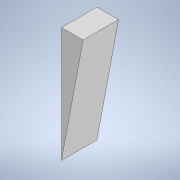
# Autodesk Inventor part: backPlateForLight
Saved by Autodesk Inventor 2021.1 (Build 251245000, 245)
## iProperties
Created: 2020-08-01
Part Number: backPlateForLight
Material: Generic
Document SubType Name: Modeling
Designer: robst
Density: 1 g/cm^3
Appearance: Default
Author: robst
Autodesk Inventor part; units mm, degrees
ref_plane "YZ Plane" through (0, 0, 0) normal (1, 0, 0) x (0, 1, 0)
ref_plane "XZ Plane" through (0, 0, 0) normal (0, 1, 0) x (-1, 0, 0)
ref_plane "XY Plane" through (0, 0, 0) normal (0, 0, 1) x (1, 0, 0)
sketch "Sketch1" plane through (0, 0, 0) normal (0, 0, 1) x (1, 0, 0)
  line L0 (0, 0) -> (0, 82.55)
  line L1 (0, 82.55) -> (15.494, 82.55)
  line L2 (15.494, 82.55) -> (0, 0)
  dimension "d0" = 82.55
  dimension "d1" = 15.494
  constraints: 6 end point, 1 perpendicular, 1 vertical
  measures "d0" distance of L0.start L0.end
  measures "d1" distance of L0.end L1.end
extrude "Extrusion1" add sketch "Sketch1" against normal blind 25.4
sketch "Sketch2" plane through (0, 0, 0) normal (-1, 0, 0) x (0, 0, 1)
  line L0 (-25.4, 82.55) -> (-25.4, 0) projected
  line L1 (-25.4, 62.641) -> (0, 62.641) construction
  line L2 (0, 0) -> (0, 82.55) projected
  line L3 (-14.8227, 65.816) -> (-17.0097, 59.466)
  line L4 (-17.0097, 59.466) -> (-17.9205, 59.466)
  line L5 (-17.9205, 59.466) -> (-20.1075, 65.816)
  line L6 (-20.1075, 65.816) -> (-19.2018, 65.816)
  line L7 (-19.2018, 65.816) -> (-17.4419, 60.5415)
  line L8 (-17.4419, 60.5415) -> (-15.682, 65.816)
  line L9 (-15.682, 65.816) -> (-14.8227, 65.816)
  spline S0 degree 2 poles (-10.3715, 62.641) (-10.3715, 60.9325) (-11.3646, 59.3322) (-12.399, 59.3322) knots 0 0 0 1 2 2 2
  spline S1 degree 2 poles (-12.399, 59.3322) (-13.4487, 59.3322) (-14.4316, 60.9634) (-14.4316, 62.6358) knots 0 0 0 1 2 2 2
  spline S2 degree 2 poles (-14.4316, 62.6358) (-14.4316, 64.3545) (-13.4384, 65.9446) (-12.399, 65.9446) knots 0 0 0 1 2 2 2
  spline S3 degree 2 poles (-12.399, 65.9446) (-11.3544, 65.9446) (-10.3715, 64.2979) (-10.3715, 62.641) knots 0 0 0 1 2 2 2
  spline S4 degree 2 poles (-11.4624, 60.7061) (-11.3389, 61.02) (-11.236, 61.9874) (-11.236, 62.641) knots 0 0 0 1 2 2 2
  spline S5 degree 2 poles (-11.236, 62.641) (-11.236, 63.2945) (-11.3389, 64.2568) (-11.4676, 64.581) knots 0 0 0 1 2 2 2
  spline S6 degree 2 poles (-11.4676, 64.581) (-11.5962, 64.9052) (-12.0439, 65.2396) (-12.399, 65.2396) knots 0 0 0 1 2 2 2
  spline S7 degree 2 poles (-12.399, 65.2396) (-12.754, 65.2396) (-13.212, 64.9052) (-13.3458, 64.5707) knots 0 0 0 1 2 2 2
  spline S8 degree 2 poles (-13.3458, 64.5707) (-13.4745, 64.2465) (-13.5671, 63.2585) (-13.5671, 62.6358) knots 0 0 0 1 2 2 2
  spline S9 degree 2 poles (-13.5671, 62.6358) (-13.5671, 61.9669) (-13.4847, 61.0715) (-13.351, 60.7216) knots 0 0 0 1 2 2 2
  spline S10 degree 2 poles (-13.351, 60.7216) (-13.2275, 60.3922) (-12.7695, 60.0372) (-12.399, 60.0372) knots 0 0 0 1 2 2 2
  spline S11 degree 2 poles (-12.399, 60.0372) (-12.049, 60.0372) (-11.5911, 60.3716) (-11.4624, 60.7061) knots 0 0 0 1 2 2 2
  line L10 (-5.9615, 59.466) -> (-9.0593, 59.466)
  line L11 (-9.0593, 59.466) -> (-9.0593, 60.1144)
  line L12 (-9.0593, 60.1144) -> (-7.9066, 60.1144)
  line L13 (-7.9066, 60.1144) -> (-7.9066, 64.37)
  line L14 (-7.9066, 64.37) -> (-9.0593, 64.37)
  line L15 (-9.0593, 64.37) -> (-9.0593, 64.9515)
  spline S12 degree 2 poles (-9.0593, 64.9515) (-8.4058, 64.9515) (-7.7883, 65.322) (-7.7471, 65.8366) knots 0 0 0 1 2 2 2
  line L16 (-7.7471, 65.8366) -> (-7.0884, 65.8366)
  line L17 (-7.0884, 65.8366) -> (-7.0884, 60.1144)
  line L18 (-7.0884, 60.1144) -> (-5.9615, 60.1144)
  line L19 (-5.9615, 60.1144) -> (-5.9615, 59.466)
  constraints: 2 end point, 2 horizontal, 2 point on line
extrude "Extrusion2" cut sketch "Sketch2" against normal blind 2.54
body "Solid1"
